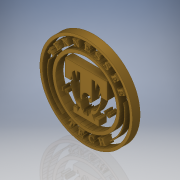
# Autodesk Inventor part: Brass Logo
Saved by Autodesk Inventor 2018 (Build 220112000, 112)
## iProperties
Created: 2017-11-28
Part Number: Brass Logo
Material: Brass, Soft Yellow
Document SubType Name: Modeling
Designer: Rus
Density: 8.47 g/cm^3
Appearance: Brass - Satin
Author: Rus
Autodesk Inventor part; units mm, degrees
(part 1 of 4)
ref_plane "YZ Plane" through (0, 0, 0) normal (1, 0, 0) x (0, 1, 0)
ref_plane "XZ Plane" through (0, 0, 0) normal (0, 1, 0) x (-1, 0, 0)
ref_plane "XY Plane" through (0, 0, 0) normal (0, 0, 1) x (1, 0, 0)
sketch "Sketch1" plane through (0, 0, 0) normal (0, 0, 1) x (1, 0, 0)
  line L0 (3.701247, -2.541841) -> (-3.701247, -2.541841)
  arc A0 (-5.715, -0.528088) -> (-3.701247, -2.541841) centre (-3.701247, -0.528088) ccw
  spline S0 degree 4 poles (-5.715, -0.528088) (-5.715, 3.281347) (0, 6.58346) (5.715, 3.281347) (5.715, -0.528088) knots -1 -1 -1 -1 -1 0 0 0 0 0
  arc A1 (3.701247, -2.541841) -> (5.715, -0.528088) centre (3.701247, -0.528088) ccw
  line L1 (9.525, -4.925915) -> (9.525, -1.750915)
  spline S1 degree 4 poles (9.525, -1.750915) (9.525, 7.774085) (0, 7.774085) (-9.525, 7.774085) (-9.525, -1.750915) knots 1 1 1 1 1 2 2 2 2 2
  line L2 (-9.525, -1.750915) -> (-9.525, -4.925915)
  arc A2 (-9.525, -4.925915) -> (9.525, -4.925915) centre (0, -45.086841) ccw
  circle A3 centre (0, -45.086841) radius 38.1
  dimension "d0" = 76.2
  constraints: 1 centre point, 1 coincident
  measures "d0" diameter of A3
extrude "Extrusion1" add sketch "Sketch1" along normal mid plane 6.35 contours A3
sketch "Sketch3" plane through (0, -45.086841, 3.175) normal (0, 0, 1) x (1, 0, 0)
  line L0 (0, -35.952322) -> (-0.919924, -35.952322)
  line L1 (-0.919924, -35.952322) -> (-3.676459, -35.766299)
  line L2 (-3.676459, -35.766299) -> (-7.246239, -35.221621)
  line L3 (-7.246239, -35.221621) -> (-10.691812, -34.335872)
  line L4 (-10.691812, -34.335872) -> (-13.995083, -33.126655)
  line L5 (-13.995083, -33.126655) -> (-17.136999, -31.612542)
  line L6 (-17.136999, -31.612542) -> (-20.101103, -29.812145)
  line L7 (-20.101103, -29.812145) -> (-22.868896, -27.741982)
  line L8 (-22.868896, -27.741982) -> (-25.421692, -25.421692)
  line L9 (-25.421692, -25.421692) -> (-27.74301, -22.868896)
  line L10 (-27.74301, -22.868896) -> (-29.812145, -20.101103)
  line L11 (-29.812145, -20.101103) -> (-31.612542, -17.136999)
  line L12 (-31.612542, -17.136999) -> (-33.126655, -13.99394)
  line L13 (-33.126655, -13.99394) -> (-34.335872, -10.690669)
  line L14 (-34.335872, -10.690669) -> (-35.221621, -7.246239)
  line L15 (-35.221621, -7.246239) -> (-35.766299, -3.67646)
  line L16 (-35.766299, -3.67646) -> (-35.951293, -0.919925)
  line L17 (-35.951293, -0.919925) -> (-35.951293, -0.001143)
  line L18 (-35.951293, -0.001143) -> (-35.951293, 0.918972)
  line L19 (-35.951293, 0.918972) -> (-35.766299, 3.675316)
  line L20 (-35.766299, 3.675316) -> (-35.221621, 7.245096)
  line L21 (-35.221621, 7.245096) -> (-34.335872, 10.689717)
  line L22 (-34.335872, 10.689717) -> (-33.126655, 13.992987)
  line L23 (-33.126655, 13.992987) -> (-31.612542, 17.136046)
  line L24 (-31.612542, 17.136046) -> (-29.812145, 20.100036)
  line L25 (-29.812145, 20.100036) -> (-27.74301, 22.868001)
  line L26 (-27.74301, 22.868001) -> (-25.421692, 25.420701)
  line L27 (-25.421692, 25.420701) -> (-22.868896, 27.740991)
  line L28 (-22.868896, 27.740991) -> (-20.101103, 29.811155)
  line L29 (-20.101103, 29.811155) -> (-17.136999, 31.61157)
  line L30 (-17.136999, 31.61157) -> (-13.995083, 33.125664)
  line L31 (-13.995083, 33.125664) -> (-10.691812, 34.334958)
  line L32 (-10.691812, 34.334958) -> (-7.246239, 35.220592)
  line L33 (-7.246239, 35.220592) -> (-3.676459, 35.765232)
  line L34 (-3.676459, 35.765232) -> (-0.919924, 35.950207)
  line L35 (-0.919924, 35.950207) -> (0, 35.950207)
  line L36 (0, 35.950207) -> (0.918972, 35.950207)
  line L37 (0.918972, 35.950207) -> (3.675317, 35.765232)
  line L38 (3.675317, 35.765232) -> (7.245096, 35.220592)
  line L39 (7.245096, 35.220592) -> (10.69067, 34.334958)
  line L40 (10.69067, 34.334958) -> (13.99413, 33.125664)
  line L41 (13.99413, 33.125664) -> (17.136999, 31.61157)
  line L42 (17.136999, 31.61157) -> (20.101179, 29.811155)
  line L43 (20.101179, 29.811155) -> (22.868954, 27.740991)
  line L44 (22.868954, 27.740991) -> (25.421653, 25.420701)
  line L45 (25.421653, 25.420701) -> (27.742134, 22.868001)
  line L46 (27.742134, 22.868001) -> (29.812107, 20.100036)
  line L47 (29.812107, 20.100036) -> (31.612332, 17.136046)
  line L48 (31.612332, 17.136046) -> (33.126617, 13.992987)
  line L49 (33.126617, 13.992987) -> (34.33572, 10.689717)
  line L50 (34.33572, 10.689717) -> (35.221545, 7.245096)
  line L51 (35.221545, 7.245096) -> (35.766375, 3.675316)
  line L52 (35.766375, 3.675316) -> (35.952303, 0.918972)
  line L53 (35.952303, 0.918972) -> (35.952303, -0.001143)
  line L54 (35.952303, -0.001143) -> (35.952303, -0.919925)
  line L55 (35.952303, -0.919925) -> (35.766375, -3.67646)
  line L56 (35.766375, -3.67646) -> (35.221545, -7.246239)
  line L57 (35.221545, -7.246239) -> (34.33572, -10.690669)
  line L58 (34.33572, -10.690669) -> (33.126617, -13.99394)
  line L59 (33.126617, -13.99394) -> (31.612332, -17.136999)
  line L60 (31.612332, -17.136999) -> (29.812107, -20.101103)
  line L61 (29.812107, -20.101103) -> (27.742134, -22.868896)
  line L62 (27.742134, -22.868896) -> (25.421653, -25.421692)
  line L63 (25.421653, -25.421692) -> (22.868954, -27.741982)
  line L64 (22.868954, -27.741982) -> (20.101179, -29.812145)
  line L65 (20.101179, -29.812145) -> (17.136999, -31.612542)
  line L66 (17.136999, -31.612542) -> (13.99413, -33.126655)
  line L67 (13.99413, -33.126655) -> (10.69067, -34.335872)
  line L68 (10.69067, -34.335872) -> (7.245096, -35.221621)
  line L69 (7.245096, -35.221621) -> (3.675317, -35.766299)
  line L70 (3.675317, -35.766299) -> (0.918972, -35.952322)
  line L71 (0.918972, -35.952322) -> (0, -35.952322)
  line L72 (0, 38.098857) -> (-0.974788, 38.098857)
  line L73 (-0.974788, 38.098857) -> (-3.896487, 37.902642)
  line L74 (-3.896487, 37.902642) -> (-7.679055, 37.325808)
  line L75 (-7.679055, 37.325808) -> (-11.330559, 36.386262)
  line L76 (-11.330559, 36.386262) -> (-14.830044, 35.104959)
  line L77 (-14.830044, 35.104959) -> (-18.161127, 33.500758)
  line L78 (-18.161127, 33.500758) -> (-21.302053, 31.592901)
  line L79 (-21.302053, 31.592901) -> (-24.235219, 29.398722)
  line L80 (-24.235219, 29.398722) -> (-26.940986, 26.939938)
  line L81 (-26.940986, 26.939938) -> (-29.399751, 24.234267)
  line L82 (-29.399751, 24.234267) -> (-31.593949, 21.301138)
  line L83 (-31.593949, 21.301138) -> (-33.501825, 18.160174)
  line L84 (-33.501825, 18.160174) -> (-35.105873, 14.829091)
  line L85 (-35.105873, 14.829091) -> (-36.387441, 11.329416)
  line L86 (-36.387441, 11.329416) -> (-37.326919, 7.678293)
  line L87 (-37.326919, 7.678293) -> (-37.903629, 3.895534)
  line L88 (-37.903629, 3.895534) -> (-38.1, 0.973645)
  line L89 (-38.1, 0.973645) -> (-38.1, -0.001143)
  line L90 (-38.1, -0.001143) -> (-38.1, -0.974789)
  line L91 (-38.1, -0.974789) -> (-37.903629, -3.896487)
  line L92 (-37.903629, -3.896487) -> (-37.326919, -7.679055)
  line L93 (-37.326919, -7.679055) -> (-36.387441, -11.329416)
  line L94 (-36.387441, -11.329416) -> (-35.105873, -14.830044)
  line L95 (-35.105873, -14.830044) -> (-33.501825, -18.161127)
  line L96 (-33.501825, -18.161127) -> (-31.593949, -21.302053)
  line L97 (-31.593949, -21.302053) -> (-29.399751, -24.23522)
  line L98 (-29.399751, -24.23522) -> (-26.940986, -26.940986)
  line L99 (-26.940986, -26.940986) -> (-24.235219, -29.399751)
  line L100 (-24.235219, -29.399751) -> (-21.302053, -31.592882)
  line L101 (-21.302053, -31.592882) -> (-18.161127, -33.500797)
  line L102 (-18.161127, -33.500797) -> (-14.830044, -35.105873)
  line L103 (-14.830044, -35.105873) -> (-11.330559, -36.386411)
  line L104 (-11.330559, -36.386411) -> (-7.679055, -37.325888)
  line L105 (-7.679055, -37.325888) -> (-3.896487, -37.902596)
  line L106 (-3.896487, -37.902596) -> (-0.974788, -38.1)
  line L107 (-0.974788, -38.1) -> (0, -38.1)
  line L108 (0, -38.1) -> (0.973645, -38.1)
  line L109 (0.973645, -38.1) -> (3.895535, -37.902596)
  line L110 (3.895535, -37.902596) -> (7.678293, -37.325888)
  line L111 (7.678293, -37.325888) -> (11.329416, -36.386411)
  line L112 (11.329416, -36.386411) -> (14.829091, -35.105873)
  line L113 (14.829091, -35.105873) -> (18.160175, -33.500797)
  line L114 (18.160175, -33.500797) -> (21.301139, -31.592882)
  line L115 (21.301139, -31.592882) -> (24.234267, -29.399751)
  line L116 (24.234267, -29.399751) -> (26.939939, -26.940986)
  line L117 (26.939939, -26.940986) -> (29.398722, -24.23522)
  line L118 (29.398722, -24.23522) -> (31.592901, -21.302053)
  line L119 (31.592901, -21.302053) -> (33.500758, -18.161127)
  line L120 (33.500758, -18.161127) -> (35.104959, -14.830044)
  line L121 (35.104959, -14.830044) -> (36.386262, -11.329416)
  line L122 (36.386262, -11.329416) -> (37.325808, -7.679055)
  line L123 (37.325808, -7.679055) -> (37.902642, -3.896487)
  line L124 (37.902642, -3.896487) -> (38.1, -0.974789)
  line L125 (38.1, -0.974789) -> (38.1, -0.001143)
  line L126 (38.1, -0.001143) -> (38.1, 0.973645)
  line L127 (38.1, 0.973645) -> (37.902642, 3.895534)
  line L128 (37.902642, 3.895534) -> (37.325808, 7.678293)
  line L129 (37.325808, 7.678293) -> (36.386262, 11.329416)
  line L130 (36.386262, 11.329416) -> (35.104959, 14.829091)
  line L131 (35.104959, 14.829091) -> (33.500758, 18.160174)
  line L132 (33.500758, 18.160174) -> (31.592901, 21.301138)
  line L133 (31.592901, 21.301138) -> (29.398722, 24.234267)
  line L134 (29.398722, 24.234267) -> (26.939939, 26.939938)
  line L135 (26.939939, 26.939938) -> (24.234267, 29.398722)
  line L136 (24.234267, 29.398722) -> (21.301139, 31.592901)
  line L137 (21.301139, 31.592901) -> (18.160175, 33.500758)
  line L138 (18.160175, 33.500758) -> (14.829091, 35.104959)
  line L139 (14.829091, 35.104959) -> (11.329416, 36.386262)
  line L140 (11.329416, 36.386262) -> (7.678293, 37.325808)
  line L141 (7.678293, 37.325808) -> (3.895535, 37.902642)
  line L142 (3.895535, 37.902642) -> (0.973645, 38.098857)
  line L143 (0.973645, 38.098857) -> (0, 38.098857)
  line L144 (0, -25.161259) -> (-1.268158, -25.161259)
  line L145 (-1.268158, -25.161259) -> (-5.071491, -24.649671)
  line L146 (-5.071491, -24.649671) -> (-9.794938, -23.183088)
  line L147 (-9.794938, -23.183088) -> (-14.068425, -20.863846)
  line L148 (-14.068425, -20.863846) -> (-17.792128, -17.791176)
  line L149 (-17.792128, -17.791176) -> (-20.864874, -14.068425)
  line L150 (-20.864874, -14.068425) -> (-23.184117, -9.793796)
  line L151 (-23.184117, -9.793796) -> (-24.6507, -5.071491)
  line L152 (-24.6507, -5.071491) -> (-25.161259, -1.268159)
  line L153 (-25.161259, -1.268159) -> (-25.161259, -0.001143)
  line L154 (-25.161259, -0.001143) -> (-25.161259, 1.267015)
  line L155 (-25.161259, 1.267015) -> (-24.6507, 5.070538)
  line L156 (-24.6507, 5.070538) -> (-23.184117, 9.793795)
  line L157 (-23.184117, 9.793795) -> (-20.864874, 14.067282)
  line L158 (-20.864874, 14.067282) -> (-17.792128, 17.791176)
  line L159 (-17.792128, 17.791176) -> (-14.068425, 20.86375)
  line L160 (-14.068425, 20.86375) -> (-9.794938, 23.183088)
  line L161 (-9.794938, 23.183088) -> (-5.071491, 24.649557)
  line L162 (-5.071491, 24.649557) -> (-1.268158, 25.160287)
  line L163 (-1.268158, 25.160287) -> (0, 25.160287)
  line L164 (0, 25.160287) -> (1.267016, 25.160287)
  line L165 (1.267016, 25.160287) -> (5.070539, 24.649557)
  line L166 (5.070539, 24.649557) -> (9.793795, 23.183088)
  line L167 (9.793795, 23.183088) -> (14.067282, 20.86375)
  line L168 (14.067282, 20.86375) -> (17.791176, 17.791176)
  line L169 (17.791176, 17.791176) -> (20.86375, 14.067282)
  line L170 (20.86375, 14.067282) -> (23.183088, 9.793795)
  line L171 (23.183088, 9.793795) -> (24.649557, 5.070538)
  line L172 (24.649557, 5.070538) -> (25.161431, 1.267015)
  line L173 (25.161431, 1.267015) -> (25.161431, -0.001143)
  line L174 (25.161431, -0.001143) -> (25.161431, -1.268159)
  line L175 (25.161431, -1.268159) -> (24.649557, -5.071491)
  line L176 (24.649557, -5.071491) -> (23.183088, -9.793796)
  line L177 (23.183088, -9.793796) -> (20.86375, -14.068425)
  line L178 (20.86375, -14.068425) -> (17.791176, -17.791176)
  line L179 (17.791176, -17.791176) -> (14.067282, -20.863846)
  line L180 (14.067282, -20.863846) -> (9.793795, -23.183088)
  line L181 (9.793795, -23.183088) -> (5.070539, -24.649671)
  line L182 (5.070539, -24.649671) -> (1.267016, -25.161259)
  line L183 (1.267016, -25.161259) -> (0, -25.161259)
  line L184 (0, 27.596211) -> (-0.705993, 27.596211)
  line L185 (-0.705993, 27.596211) -> (-2.822638, 27.454669)
  line L186 (-2.822638, 27.454669) -> (-5.562409, 27.036141)
  line L187 (-5.562409, 27.036141) -> (-8.207311, 26.355866)
  line L188 (-8.207311, 26.355866) -> (-10.742676, 25.427749)
  line L189 (-10.742676, 25.427749) -> (-13.154787, 24.266271)
  line L190 (-13.154787, 24.266271) -> (-15.4305, 22.883241)
  line L191 (-15.4305, 22.883241) -> (-17.554575, 21.294661)
  line L192 (-17.554575, 21.294661) -> (-19.515087, 19.514058)
  line L193 (-19.515087, 19.514058) -> (-21.295862, 17.553432)
  line L194 (-21.295862, 17.553432) -> (-22.884403, 15.429357)
  line L195 (-22.884403, 15.429357) -> (-24.267243, 13.153834)
  line L196 (-24.267243, 13.153834) -> (-25.42895, 10.741533)
  line L197 (-25.42895, 10.741533) -> (-26.357047, 8.206359)
  line L198 (-26.357047, 8.206359) -> (-27.037113, 5.561457)
  line L199 (-27.037113, 5.561457) -> (-27.455679, 2.821495)
  line L200 (-27.455679, 2.821495) -> (-27.597278, 0.70485)
  line L201 (-27.597278, 0.70485) -> (-27.597278, -0.001143)
  line L202 (-27.597278, -0.001143) -> (-27.597278, -0.705993)
  line L203 (-27.597278, -0.705993) -> (-27.455679, -2.821496)
  line L204 (-27.455679, -2.821496) -> (-27.037113, -5.56241)
  line L205 (-27.037113, -5.56241) -> (-26.357047, -8.206359)
  line L206 (-26.357047, -8.206359) -> (-25.42895, -10.742676)
  line L207 (-25.42895, -10.742676) -> (-24.267243, -13.154787)
  line L208 (-24.267243, -13.154787) -> (-22.884403, -15.429547)
  line L209 (-22.884403, -15.429547) -> (-21.295862, -17.554575)
  line L210 (-21.295862, -17.554575) -> (-19.515087, -19.514058)
  line L211 (-19.515087, -19.514058) -> (-17.554575, -21.294833)
  line L212 (-17.554575, -21.294833) -> (-15.4305, -22.883355)
  line L213 (-15.4305, -22.883355) -> (-13.154787, -24.266214)
  line L214 (-13.154787, -24.266214) -> (-10.742676, -25.427921)
  line L215 (-10.742676, -25.427921) -> (-8.207311, -26.356018)
  line L216 (-8.207311, -26.356018) -> (-5.562409, -27.036084)
  line L217 (-5.562409, -27.036084) -> (-2.822638, -27.45465)
  line L218 (-2.822638, -27.45465) -> (-0.705993, -27.597278)
  line L219 (-0.705993, -27.597278) -> (0, -27.597278)
  line L220 (0, -27.597278) -> (0.70485, -27.597278)
  line L221 (0.70485, -27.597278) -> (2.821496, -27.45465)
  line L222 (2.821496, -27.45465) -> (5.561457, -27.036084)
  line L223 (5.561457, -27.036084) -> (8.206359, -26.356018)
  line L224 (8.206359, -26.356018) -> (10.741533, -25.427921)
  line L225 (10.741533, -25.427921) -> (13.153835, -24.266214)
  line L226 (13.153835, -24.266214) -> (15.429357, -22.883355)
  line L227 (15.429357, -22.883355) -> (17.553432, -21.294833)
  line L228 (17.553432, -21.294833) -> (19.514058, -19.514058)
  line L229 (19.514058, -19.514058) -> (21.294662, -17.554575)
  line L230 (21.294662, -17.554575) -> (22.883241, -15.429547)
  line L231 (22.883241, -15.429547) -> (24.266271, -13.154787)
  line L232 (24.266271, -13.154787) -> (25.42775, -10.742676)
  line L233 (25.42775, -10.742676) -> (26.355866, -8.206359)
  line L234 (26.355866, -8.206359) -> (27.036141, -5.56241)
  line L235 (27.036141, -5.56241) -> (27.454669, -2.821496)
  line L236 (27.454669, -2.821496) -> (27.597354, -0.705993)
  line L237 (27.597354, -0.705993) -> (27.597354, -0.001143)
  line L238 (27.597354, -0.001143) -> (27.597354, 0.70485)
  line L239 (27.597354, 0.70485) -> (27.454669, 2.821495)
  line L240 (27.454669, 2.821495) -> (27.036141, 5.561457)
  line L241 (27.036141, 5.561457) -> (26.355866, 8.206359)
  line L242 (26.355866, 8.206359) -> (25.42775, 10.741533)
  line L243 (25.42775, 10.741533) -> (24.266271, 13.153834)
  line L244 (24.266271, 13.153834) -> (22.883241, 15.429357)
  line L245 (22.883241, 15.429357) -> (21.294662, 17.553432)
  line L246 (21.294662, 17.553432) -> (19.514058, 19.514058)
  line L247 (19.514058, 19.514058) -> (17.553432, 21.294661)
  line L248 (17.553432, 21.294661) -> (15.429357, 22.883241)
  line L249 (15.429357, 22.883241) -> (13.153835, 24.266271)
  line L250 (13.153835, 24.266271) -> (10.741533, 25.427749)
  line L251 (10.741533, 25.427749) -> (8.206359, 26.355866)
  line L252 (8.206359, 26.355866) -> (5.561457, 27.036141)
  line L253 (5.561457, 27.036141) -> (2.821496, 27.454669)
  line L254 (2.821496, 27.454669) -> (0.70485, 27.596211)
  line L255 (0.70485, 27.596211) -> (0, 27.596211)
  line L256 (17.172051, 16.11268) -> (17.172051, 2.422588)
  line L257 (17.172051, 2.422588) -> (12.363259, 2.422588)
  line L258 (12.363259, 2.422588) -> (12.363259, 2.817304)
  line L259 (12.363259, 2.817304) -> (12.3063, 3.999738)
  line L260 (12.3063, 3.999738) -> (12.175045, 5.195697)
  line L261 (12.175045, 5.195697) -> (12.137708, 5.418582)
  line L262 (12.137708, 5.418582) -> (9.773222, 1.311592)
  line L263 (9.773222, 1.311592) -> (11.41838, 8.127682)
  line L264 (11.41838, 8.127682) -> (11.292459, 8.4201)
  line L265 (11.292459, 8.4201) -> (10.479786, 9.628441)
  line L266 (10.479786, 9.628441) -> (9.415463, 10.516171)
  line L267 (9.415463, 10.516171) -> (9.16324, 10.648378)
  line L268 (9.16324, 10.648378) -> (7.332916, 4.981575)
  line L269 (7.332916, 4.981575) -> (7.258621, 11.266551)
  line L270 (7.258621, 11.266551) -> (7.070407, 11.299507)
  line L271 (7.070407, 11.299507) -> (6.058472, 11.397805)
  line L272 (6.058472, 11.397805) -> (4.950524, 11.415522)
  line L273 (4.950524, 11.415522) -> (4.714875, 11.406949)
  line L274 (4.714875, 11.406949) -> (4.725162, -4.028885)
  line L275 (4.725162, -4.028885) -> (4.725162, -4.259199)
  line L276 (4.725162, -4.259199) -> (4.528947, -4.953762)
  line L277 (4.528947, -4.953762) -> (4.022408, -5.571935)
  line L278 (4.022408, -5.571935) -> (3.332226, -5.801296)
  line L279 (3.332226, -5.801296) -> (2.736914, -5.668899)
  line L280 (2.736914, -5.668899) -> (2.579751, -5.564505)
  line L281 (2.579751, -5.564505) -> (2.432876, -5.466207)
  line L282 (2.432876, -5.466207) -> (2.098167, -5.013579)
  line L283 (2.098167, -5.013579) -> (1.903667, -4.272534)
  line L284 (1.903667, -4.272534) -> (2.051495, -3.487293)
  line L285 (2.051495, -3.487293) -> (2.427732, -2.934272)
  line L286 (2.427732, -2.934272) -> (2.596325, -2.805875)
  line L287 (2.596325, -2.805875) -> (3.382709, -2.657285)
  line L288 (3.382709, -2.657285) -> (3.809429, -2.90322)
  line L289 (3.809429, -2.90322) -> (3.837432, -2.702624)
  line L290 (3.837432, -2.702624) -> (3.792093, -2.084642)
  line L291 (3.792093, -2.084642) -> (3.49758, -1.562672)
  line L292 (3.49758, -1.562672) -> (2.978658, -1.279589)
  line L293 (2.978658, -1.279589) -> (2.462022, -1.185291)
  line L294 (2.462022, -1.185291) -> (2.289239, -1.179195)
  line L295 (2.289239, -1.179195) -> (2.020633, -1.011746)
  line L296 (2.020633, -1.011746) -> (1.109853, -0.676085)
  line L297 (1.109853, -0.676085) -> (-0.02267, -0.608838)
  line L298 (-0.02267, -0.608838) -> (-1.061466, -0.920687)
  line L299 (-1.061466, -0.920687) -> (-1.959483, -1.555433)
  line L300 (-1.959483, -1.555433) -> (-2.670619, -2.454593)
  line L301 (-2.670619, -2.454593) -> (-3.148012, -3.562541)
  line L302 (-3.148012, -3.562541) -> (-3.344608, -4.820412)
  line L303 (-3.344608, -4.820412) -> (-3.287649, -5.843588)
  line L304 (-3.287649, -5.843588) -> (-3.213354, -6.1722)
  line L305 (-3.213354, -6.1722) -> (-3.182112, -6.310884)
  line L306 (-3.182112, -6.310884) -> (-3.203829, -6.785229)
  line L307 (-3.203829, -6.785229) -> (-3.458146, -7.027926)
  line L308 (-3.458146, -7.027926) -> (-3.54311, -7.050596)
  line L309 (-3.54311, -7.050596) -> (-3.686746, -7.087934)
  line L310 (-3.686746, -7.087934) -> (-4.161854, -7.030974)
  line L311 (-4.161854, -7.030974) -> (-4.604194, -6.670358)
  line L312 (-4.604194, -6.670358) -> (-4.868799, -6.078284)
  line L313 (-4.868799, -6.078284) -> (-4.95662, -5.54374)
  line L314 (-4.95662, -5.54374) -> (-4.95662, -5.366004)
  line L315 (-4.95662, -5.366004) -> (-4.946332, 11.406949)
  line L316 (-4.946332, 11.406949) -> (-5.183124, 11.415522)
  line L317 (-5.183124, 11.415522) -> (-6.291072, 11.397805)
  line L318 (-6.291072, 11.397805) -> (-7.302055, 11.298555)
  line L319 (-7.302055, 11.298555) -> (-7.490079, 11.265408)
  line L320 (-7.490079, 11.265408) -> (-7.564374, 4.981575)
  line L321 (-7.564374, 4.981575) -> (-9.394889, 10.648378)
  line L322 (-9.394889, 10.648378) -> (-9.64692, 10.516171)
  line L323 (-9.64692, 10.516171) -> (-10.711434, 9.628441)
  line L324 (-10.711434, 9.628441) -> (-11.522964, 8.418957)
  line L325 (-11.522964, 8.418957) -> (-11.648884, 8.12673)
  line L326 (-11.648884, 8.12673) -> (-10.004488, 1.311592)
  line L327 (-10.004488, 1.311592) -> (-12.356782, 5.399151)
  line L328 (-12.356782, 5.399151) -> (-12.395073, 5.176837)
  line L329 (-12.395073, 5.176837) -> (-12.528423, 3.988308)
  line L330 (-12.528423, 3.988308) -> (-12.584239, 2.814447)
  line L331 (-12.584239, 2.814447) -> (-12.584239, 2.422588)
  line L332 (-12.584239, 2.422588) -> (-17.341596, 2.422588)
  line L333 (-17.341596, 2.422588) -> (-17.341596, 16.11268)
  line L334 (-17.341596, 16.11268) -> (17.172051, 16.11268)
  line L335 (1.435608, -12.052935) -> (2.963037, -14.304074)
  line L336 (2.963037, -14.304074) -> (3.054096, -14.131481)
  line L337 (3.054096, -14.131481) -> (3.477959, -13.134022)
  line L338 (3.477959, -13.134022) -> (3.854958, -11.942445)
  line L339 (3.854958, -11.942445) -> (3.923157, -11.673649)
  line L340 (3.923157, -11.673649) -> (4.728401, -9.001125)
  line L341 (4.728401, -9.001125) -> (4.776978, -9.177528)
  line L342 (4.776978, -9.177528) -> (5.028057, -9.683305)
  line L343 (5.028057, -9.683305) -> (5.437442, -10.062401)
  line L344 (5.437442, -10.062401) -> (5.922074, -10.187559)
  line L345 (5.922074, -10.187559) -> (6.446139, -10.110026)
  line L346 (6.446139, -10.110026) -> (6.974205, -9.877425)
  line L347 (6.974205, -9.877425) -> (7.470267, -9.540621)
  line L348 (7.470267, -9.540621) -> (7.900225, -9.149906)
  line L349 (7.900225, -9.149906) -> (8.155495, -8.85825)
  line L350 (8.155495, -8.85825) -> (8.229029, -8.754047)
  line L351 (8.229029, -8.754047) -> (8.690039, -8.088249)
  line L352 (8.690039, -8.088249) -> (9.885616, -5.960174)
  line L353 (9.885616, -5.960174) -> (11.095101, -3.139821)
  line L354 (11.095101, -3.139821) -> (11.871008, -0.474345)
  line L355 (11.871008, -0.474345) -> (12.186475, 1.269111)
  line L356 (12.186475, 1.269111) -> (12.228766, 1.854136)
  line L357 (12.228766, 1.854136) -> (12.233719, 1.745742)
  line L358 (12.233719, 1.745742) -> (12.257532, 0.599503)
  line L359 (12.257532, 0.599503) -> (12.257532, 0.478726)
  line L360 (12.257532, 0.478726) -> (12.255437, -0.115634)
  line L361 (12.255437, -0.115634) -> (12.008549, -1.901571)
  line L362 (12.008549, -1.901571) -> (11.267504, -4.741926)
  line L363 (11.267504, -4.741926) -> (10.014014, -7.805166)
  line L364 (10.014014, -7.805166) -> (8.731187, -10.131743)
  line L365 (8.731187, -10.131743) -> (8.229029, -10.856024)
  line L366 (8.229029, -10.856024) -> (8.162925, -10.950321)
  line L367 (8.162925, -10.950321) -> (7.954137, -11.226356)
  line L368 (7.954137, -11.226356) -> (7.590282, -11.667554)
  line L369 (7.590282, -11.667554) -> (7.162228, -12.131611)
  line L370 (7.162228, -12.131611) -> (6.693217, -12.57281)
  line L371 (6.693217, -12.57281) -> (6.208395, -12.941808)
  line L372 (6.208395, -12.941808) -> (5.731955, -13.193078)
  line L373 (5.731955, -13.193078) -> (5.287518, -13.278802)
  line L374 (5.287518, -13.278802) -> (4.978337, -13.207555)
  line L375 (4.978337, -13.207555) -> (4.900041, -13.151739)
  line L376 (4.900041, -13.151739) -> (4.910328, -13.227177)
  line L377 (4.910328, -13.227177) -> (5.110734, -13.861732)
  line L378 (5.110734, -13.861732) -> (5.144834, -13.927836)
  line L379 (5.144834, -13.927836) -> (6.803707, -17.177195)
  line L380 (6.803707, -17.177195) -> (6.803707, -14.610017)
  line L381 (6.803707, -14.610017) -> (6.829615, -14.613065)
  line L382 (6.829615, -14.613065) -> (7.101459, -14.645069)
  line L383 (7.101459, -14.645069) -> (7.130224, -14.648117)
  line L384 (7.130224, -14.648117) -> (7.284339, -14.665833)
  line L385 (7.284339, -14.665833) -> (8.410765, -14.740128)
  line L386 (8.410765, -14.740128) -> (10.014966, -14.79804)
  line L387 (10.014966, -14.79804) -> (10.407586, -14.807375)
  line L388 (10.407586, -14.807375) -> (10.407586, -19.352819)
  line L389 (10.407586, -19.352819) -> (-10.628757, -19.352819)
  line L390 (-10.628757, -19.352819) -> (-10.628757, -14.807375)
  line L391 (-10.628757, -14.807375) -> (-10.244328, -14.807375)
  line L392 (-10.244328, -14.807375) -> (-9.089707, -14.779371)
  line L393 (-9.089707, -14.779371) -> (-7.975854, -14.712315)
  line L394 (-7.975854, -14.712315) -> (-7.775257, -14.692694)
  line L395 (-7.775257, -14.692694) -> (-7.705915, -14.685454)
  line L396 (-7.705915, -14.685454) -> (-7.051738, -14.602778)
  line L397 (-7.051738, -14.602778) -> (-6.990779, -14.593443)
  line L398 (-6.990779, -14.593443) -> (-6.990779, -17.177195)
  line L399 (-6.990779, -17.177195) -> (-5.38372, -14.030135)
  line L400 (-5.38372, -14.030135) -> (-5.346383, -13.955649)
  line L401 (-5.346383, -13.955649) -> (-5.071491, -13.174409)
  line L402 (-5.071491, -13.174409) -> (-5.060061, -13.094779)
  line L403 (-5.060061, -13.094779) -> (-5.134546, -13.162026)
  line L404 (-5.134546, -13.162026) -> (-5.443537, -13.272516)
  line L405 (-5.443537, -13.272516) -> (-5.892355, -13.217843)
  line L406 (-5.892355, -13.217843) -> (-6.377749, -12.982194)
  line L407 (-6.377749, -12.982194) -> (-6.874955, -12.614148)
  line L408 (-6.874955, -12.614148) -> (-7.358634, -12.167807)
  line L409 (-7.358634, -12.167807) -> (-7.802118, -11.691366)
  line L410 (-7.802118, -11.691366) -> (-8.177212, -11.236642)
  line L411 (-8.177212, -11.236642) -> (-8.392287, -10.953179)
  line L412 (-8.392287, -10.953179) -> (-8.459533, -10.856024)
  line L413 (-8.459533, -10.856024) -> (-8.961691, -10.131743)
  line L414 (-8.961691, -10.131743) -> (-10.245471, -7.805166)
  line L415 (-10.245471, -7.805166) -> (-11.498961, -4.741926)
  line L416 (-11.498961, -4.741926) -> (-12.241149, -1.901571)
  line L417 (-12.241149, -1.901571) -> (-12.487084, -0.115634)
  line L418 (-12.487084, -0.115634) -> (-12.48918, 0.478726)
  line L419 (-12.48918, 0.478726) -> (-12.490132, 0.599503)
  line L420 (-12.490132, 0.599503) -> (-12.465367, 1.745742)
  line L421 (-12.465367, 1.745742) -> (-12.459081, 1.854136)
  line L422 (-12.459081, 1.854136) -> (-12.41679, 1.269111)
  line L423 (-12.41679, 1.269111) -> (-12.102655, -0.474345)
  line L424 (-12.102655, -0.474345) -> (-11.326558, -3.139821)
  line L425 (-11.326558, -3.139821) -> (-10.117074, -5.960174)
  line L426 (-10.117074, -5.960174) -> (-8.921496, -8.088249)
  line L427 (-8.921496, -8.088249) -> (-8.459533, -8.754047)
  line L428 (-8.459533, -8.754047) -> (-8.386953, -8.85825)
  line L429 (-8.386953, -8.85825) -> (-8.132826, -9.149906)
  line L430 (-8.132826, -9.149906) -> (-7.702867, -9.540621)
  line L431 (-7.702867, -9.540621) -> (-7.205662, -9.877425)
  line L432 (-7.205662, -9.877425) -> (-6.678549, -10.110026)
  line L433 (-6.678549, -10.110026) -> (-6.154674, -10.187559)
  line L434 (-6.154674, -10.187559) -> (-5.670042, -10.062401)
  line L435 (-5.670042, -10.062401) -> (-5.259705, -9.683305)
  line L436 (-5.259705, -9.683305) -> (-5.007483, -9.178671)
  line L437 (-5.007483, -9.178671) -> (-4.958905, -9.001125)
  line L438 (-4.958905, -9.001125) -> (-4.153662, -11.673649)
  line L439 (-4.153662, -11.673649) -> (-4.082605, -11.956923)
  line L440 (-4.082605, -11.956923) -> (-3.681412, -13.206412)
  line L441 (-3.681412, -13.206412) -> (-3.227641, -14.241018)
  line L442 (-3.227641, -14.241018) -> (-3.129534, -14.417802)
  line L443 (-3.129534, -14.417802) -> (-1.523429, -12.052935)
  line L444 (-1.523429, -12.052935) -> (-2.357437, -15.50289)
  line L445 (-2.357437, -15.50289) -> (-2.234375, -15.635288)
  line L446 (-2.234375, -15.635288) -> (-1.584388, -16.134398)
  line L447 (-1.584388, -16.134398) -> (-0.900112, -16.433102)
  line L448 (-0.900112, -16.433102) -> (-0.758571, -16.465106)
  line L449 (-0.758571, -16.465106) -> (-0.027813, -12.36726)
  line L450 (-0.027813, -12.36726) -> (0.783336, -16.399002)
  line L451 (0.783336, -16.399002) -> (0.911543, -16.356711)
  line L452 (0.911543, -16.356711) -> (1.534859, -16.02486)
  line L453 (1.534859, -16.02486) -> (2.126933, -15.51432)
  line L454 (2.126933, -15.51432) -> (2.240661, -15.384018)
  line L455 (2.240661, -15.384018) -> (1.435608, -12.052935)
  line L456 (14.425803, -8.89235) -> (14.425803, -8.548497)
  line L457 (14.425803, -8.548497) -> (14.641068, -8.548497)
  line L458 (14.641068, -8.548497) -> (14.717458, -8.548497)
  line L459 (14.717458, -8.548497) -> (14.938629, -8.50392)
  line L460 (14.938629, -8.50392) -> (14.950059, -8.495538)
  line L461 (14.950059, -8.495538) -> (14.960346, -8.486203)
  line L462 (14.960346, -8.486203) -> (15.014067, -8.32085)
  line L463 (15.014067, -8.32085) -> (15.014067, -8.266176)
  line L464 (15.014067, -8.266176) -> (15.014067, -6.736461)
  line L465 (15.014067, -6.736461) -> (14.425803, -6.736461)
  line L466 (14.425803, -6.736461) -> (14.425803, -6.397562)
  line L467 (14.425803, -6.397562) -> (14.482763, -6.394514)
  line L468 (14.482763, -6.394514) -> (14.93158, -6.296216)
  line L469 (14.93158, -6.296216) -> (14.963585, -6.279642)
  line L470 (14.963585, -6.279642) -> (14.994445, -6.262116)
  line L471 (14.994445, -6.262116) -> (15.239428, -5.990463)
  line L472 (15.239428, -5.990463) -> (15.256954, -5.953125)
  line L473 (15.256954, -5.953125) -> (15.645575, -5.953125)
  line L474 (15.645575, -5.953125) -> (15.645575, -8.27532)
  line L475 (15.645575, -8.27532) -> (15.645575, -8.331136)
  line L476 (15.645575, -8.331136) -> (15.689009, -8.492681)
  line L477 (15.689009, -8.492681) -> (15.698343, -8.500872)
  line L478 (15.698343, -8.500872) -> (15.706535, -8.507921)
  line L479 (15.706535, -8.507921) -> (15.911322, -8.548497)
  line L480 (15.911322, -8.548497) -> (15.979521, -8.548497)
  line L481 (15.979521, -8.548497) -> (16.223171, -8.548497)
  line L482 (16.223171, -8.548497) -> (16.223171, -8.89235)
  line L483 (16.223171, -8.89235) -> (14.425803, -8.89235)
  line L484 (17.692878, -8.441817) -> (17.713643, -8.458391)
  line L485 (17.713643, -8.458391) -> (17.947196, -8.584311)
  line L486 (17.947196, -8.584311) -> (17.973104, -8.593646)
  line L487 (17.973104, -8.593646) -> (17.997678, -8.602218)
  line L488 (17.997678, -8.602218) -> (18.224183, -8.643366)
  line L489 (18.224183, -8.643366) -> (18.299621, -8.643366)
  line L490 (18.299621, -8.643366) -> (18.432018, -8.643366)
  line L491 (18.432018, -8.643366) -> (18.798921, -8.484108)
  line L492 (18.798921, -8.484108) -> (18.830925, -8.452104)
  line L493 (18.830925, -8.452104) -> (18.861977, -8.4201)
  line L494 (18.861977, -8.4201) -> (19.021235, -8.041957)
  line L495 (19.021235, -8.041957) -> (19.021235, -7.915846)
  line L496 (19.021235, -7.915846) -> (19.021235, -7.777353)
  line L497 (19.021235, -7.777353) -> (18.868263, -7.395972)
  line L498 (18.868263, -7.395972) -> (18.838164, -7.363968)
  line L499 (18.838164, -7.363968) -> (18.807113, -7.330821)
  line L500 (18.807113, -7.330821) -> (18.447639, -7.16642)
  line L501 (18.447639, -7.16642) -> (18.327624, -7.16642)
  line L502 (18.327624, -7.16642) -> (18.244947, -7.16642)
  line L503 (18.244947, -7.16642) -> (18.024729, -7.228332)
  line L504 (18.024729, -7.228332) -> (17.999964, -7.241858)
  line L505 (17.999964, -7.241858) -> (17.975199, -7.254431)
  line L506 (17.975199, -7.254431) -> (17.742789, -7.445692)
  line L507 (17.742789, -7.445692) -> (17.721072, -7.472363)
  line L508 (17.721072, -7.472363) -> (17.39627, -7.457885)
  line L509 (17.39627, -7.457885) -> (17.544288, -5.909691)
  line L510 (17.544288, -5.909691) -> (17.583341, -5.922264)
  line L511 (17.583341, -5.922264) -> (17.984534, -6.018276)
  line L512 (17.984534, -6.018276) -> (18.025872, -6.024563)
  line L513 (18.025872, -6.024563) -> (18.066068, -6.030659)
  line L514 (18.066068, -6.030659) -> (18.423636, -6.062663)
  line L515 (18.423636, -6.062663) -> (18.543651, -6.062663)
  line L516 (18.543651, -6.062663) -> (18.677953, -6.062663)
  line L517 (18.677953, -6.062663) -> (19.03857, -6.031611)
  line L518 (19.03857, -6.031611) -> (19.082004, -6.025325)
  line L519 (19.082004, -6.025325) -> (19.124295, -6.019229)
  line L520 (19.124295, -6.019229) -> (19.536918, -5.927217)
  line L521 (19.536918, -5.927217) -> (19.575971, -5.914835)
  line L522 (19.575971, -5.914835) -> (19.559588, -5.972747)
  line L523 (19.559588, -5.972747) -> (19.23288, -6.401562)
  line L524 (19.23288, -6.401562) -> (19.18335, -6.429566)
  line L525 (19.18335, -6.429566) -> (19.13363, -6.457378)
  line L526 (19.13363, -6.457378) -> (18.564225, -6.597968)
  line L527 (18.564225, -6.597968) -> (18.375059, -6.597968)
  line L528 (18.375059, -6.597968) -> (18.320195, -6.597968)
  line L529 (18.320195, -6.597968) -> (18.178653, -6.588633)
  line L530 (18.178653, -6.588633) -> (18.159222, -6.587681)
  line L531 (18.159222, -6.587681) -> (18.138458, -6.585776)
  line L532 (18.138458, -6.585776) -> (17.879949, -6.555486)
  line L533 (17.879949, -6.555486) -> (17.849088, -6.551676)
  line L534 (17.849088, -6.551676) -> (17.81175, -6.989826)
  line L535 (17.81175, -6.989826) -> (17.842992, -6.975158)
  line L536 (17.842992, -6.975158) -> (18.15103, -6.867716)
  line L537 (18.15103, -6.867716) -> (18.181892, -6.860667)
  line L538 (18.181892, -6.860667) -> (18.2118, -6.853238)
  line L539 (18.2118, -6.853238) -> (18.462879, -6.818376)
  line L540 (18.462879, -6.818376) -> (18.547842, -6.818376)
  line L541 (18.547842, -6.818376) -> (18.758345, -6.818376)
  line L542 (18.758345, -6.818376) -> (19.337274, -7.062026)
  line L543 (19.337274, -7.062026) -> (19.393091, -7.111746)
  line L544 (19.393091, -7.111746) -> (19.447955, -7.160133)
  line L545 (19.447955, -7.160133) -> (19.723799, -7.678293)
  line L546 (19.723799, -7.678293) -> (19.723799, -7.851839)
  line L547 (19.723799, -7.851839) -> (19.723799, -7.967472)
  line L548 (19.723799, -7.967472) -> (19.639979, -8.315896)
  line L549 (19.639979, -8.315896) -> (19.444716, -8.621649)
  line L550 (19.444716, -8.621649) -> (19.3889, -8.672322)
  line L551 (19.3889, -8.672322) -> (19.333083, -8.722042)
  line L552 (19.333083, -8.722042) -> (18.992088, -8.897684)
  line L553 (18.992088, -8.897684) -> (18.601563, -8.974074)
  line L554 (18.601563, -8.974074) -> (18.471452, -8.974074)
  line L555 (18.471452, -8.974074) -> (18.253139, -8.974074)
  line L556 (18.253139, -8.974074) -> (17.655731, -8.786051)
  line L557 (17.655731, -8.786051) -> (17.600866, -8.748712)
  line L558 (17.600866, -8.748712) -> (17.545241, -8.710613)
  line L559 (17.545241, -8.710613) -> (17.267301, -8.30561)
  line L560 (17.267301, -8.30561) -> (17.267301, -8.171116)
  line L561 (17.267301, -8.171116) -> (17.267301, -8.093583)
  line L562 (17.267301, -8.093583) -> (17.370361, -7.884795)
  line L563 (17.370361, -7.884795) -> (17.391126, -7.864221)
  line L564 (17.391126, -7.864221) -> (17.410938, -7.843647)
  line L565 (17.410938, -7.843647) -> (17.625822, -7.740205)
  line L566 (17.625822, -7.740205) -> (17.698212, -7.740205)
  line L567 (17.698212, -7.740205) -> (17.769459, -7.740205)
  line L568 (17.769459, -7.740205) -> (17.964722, -7.819835)
  line L569 (17.964722, -7.819835) -> (17.983391, -7.836217)
  line L570 (17.983391, -7.836217) -> (18.00206, -7.851839)
  line L571 (18.00206, -7.851839) -> (18.094071, -8.026337)
  line L572 (18.094071, -8.026337) -> (18.094071, -8.085391)
  line L573 (18.094071, -8.085391) -> (18.094071, -8.150542)
  line L574 (18.094071, -8.150542) -> (18.003012, -8.329041)
  line L575 (18.003012, -8.329041) -> (17.985677, -8.345805)
  line L576 (17.985677, -8.345805) -> (17.966817, -8.361426)
  line L577 (17.966817, -8.361426) -> (17.761268, -8.441817)
  line L578 (17.761268, -8.441817) -> (17.692878, -8.441817)
  line L579 (-20.470063, -8.89235) -> (-20.470063, -8.548497)
  line L580 (-20.470063, -8.548497) -> (-20.256132, -8.548497)
  line L581 (-20.256132, -8.548497) -> (-20.179646, -8.548497)
  line L582 (-20.179646, -8.548497) -> (-19.958475, -8.50392)
  line L583 (-19.958475, -8.50392) -> (-19.947103, -8.495538)
  line L584 (-19.947103, -8.495538) -> (-19.936777, -8.486203)
  line L585 (-19.936777, -8.486203) -> (-19.88199, -8.32085)
  line L586 (-19.88199, -8.32085) -> (-19.88199, -8.266176)
  line L587 (-19.88199, -8.266176) -> (-19.88199, -6.736461)
  line L588 (-19.88199, -6.736461) -> (-20.470063, -6.736461)
  line L589 (-20.470063, -6.736461) -> (-20.470063, -6.397562)
  line L590 (-20.470063, -6.397562) -> (-20.413218, -6.394514)
  line L591 (-20.413218, -6.394514) -> (-19.965695, -6.296216)
  line L592 (-19.965695, -6.296216) -> (-19.933653, -6.279642)
  line L593 (-19.933653, -6.279642) -> (-19.901611, -6.262116)
  line L594 (-19.901611, -6.262116) -> (-19.656685, -5.990463)
  line L595 (-19.656685, -5.990463) -> (-19.639121, -5.953125)
  line L596 (-19.639121, -5.953125) -> (-19.25153, -5.953125)
  line L597 (-19.25153, -5.953125) -> (-19.25153, -8.27532)
  line L598 (-19.25153, -8.27532) -> (-19.25153, -8.331136)
  line L599 (-19.25153, -8.331136) -> (-19.207086, -8.492681)
  line L600 (-19.207086, -8.492681) -> (-19.19779, -8.500872)
  line L601 (-19.19779, -8.500872) -> (-19.189522, -8.507921)
  line L602 (-19.189522, -8.507921) -> (-18.985992, -8.548497)
  line L603 (-18.985992, -8.548497) -> (-18.917793, -8.548497)
  line L604 (-18.917793, -8.548497) -> (-18.67281, -8.548497)
  line L605 (-18.67281, -8.548497) -> (-18.67281, -8.89235)
  line L606 (-18.67281, -8.89235) -> (-20.470063, -8.89235)
  line L607 (-16.940593, -8.581454) -> (-16.926115, -8.590788)
  line L608 (-16.926115, -8.590788) -> (-16.77943, -8.658987)
  line L609 (-16.77943, -8.658987) -> (-16.763809, -8.664131)
  line L610 (-16.763809, -8.664131) -> (-16.749331, -8.668322)
  line L611 (-16.749331, -8.668322) -> (-16.617124, -8.692134)
  line L612 (-16.617124, -8.692134) -> (-16.572547, -8.692134)
  line L613 (-16.572547, -8.692134) -> (-16.441293, -8.692134)
  line L614 (-16.441293, -8.692134) -> (-16.076485, -8.464486)
  line L615 (-16.076485, -8.464486) -> (-16.047529, -8.4201)
  line L616 (-16.047529, -8.4201) -> (-16.019716, -8.37457)
  line L617 (-16.019716, -8.37457) -> (-15.871888, -7.672959)
  line L618 (-15.871888, -7.672959) -> (-15.870936, -7.579043)
  line L619 (-15.870936, -7.579043) -> (-15.900844, -7.601521)
  line L620 (-15.900844, -7.601521) -> (-16.206787, -7.771067)
  line L621 (-16.206787, -7.771067) -> (-16.237839, -7.782496)
  line L622 (-16.237839, -7.782496) -> (-16.2687, -7.793736)
  line L623 (-16.2687, -7.793736) -> (-16.544734, -7.850695)
  line L624 (-16.544734, -7.850695) -> (-16.635603, -7.850695)
  line L625 (-16.635603, -7.850695) -> (-16.81753, -7.850695)
  line L626 (-16.81753, -7.850695) -> (-17.314735, -7.627429)
  line L627 (-17.314735, -7.627429) -> (-17.36217, -7.583043)
  line L628 (-17.36217, -7.583043) -> (-17.410747, -7.538466)
  line L629 (-17.410747, -7.538466) -> (-17.653635, -7.076504)
  line L630 (-17.653635, -7.076504) -> (-17.653635, -6.92258)
  line L631 (-17.653635, -6.92258) -> (-17.653635, -6.736461)
  line L632 (-17.653635, -6.736461) -> (-17.375695, -6.225921)
  line L633 (-17.375695, -6.225921) -> (-17.319879, -6.179439)
  line L634 (-17.319879, -6.179439) -> (-17.265015, -6.132957)
  line L635 (-17.265015, -6.132957) -> (-16.638841, -5.900547)
  line L636 (-16.638841, -5.900547) -> (-16.430053, -5.900547)
  line L637 (-16.430053, -5.900547) -> (-16.294608, -5.900547)
  line L638 (-16.294608, -5.900547) -> (-15.886366, -5.997512)
  line L639 (-15.886366, -5.997512) -> (-15.536989, -6.225921)
  line L640 (-15.536989, -6.225921) -> (-15.480221, -6.291072)
  line L641 (-15.480221, -6.291072) -> (-15.424404, -6.356033)
  line L642 (-15.424404, -6.356033) -> (-15.229141, -6.761416)
  line L643 (-15.229141, -6.761416) -> (-15.144369, -7.233666)
  line L644 (-15.144369, -7.233666) -> (-15.144369, -7.39159)
  line L645 (-15.144369, -7.39159) -> (-15.144369, -7.556945)
  line L646 (-15.144369, -7.556945) -> (-15.238285, -8.053197)
  line L647 (-15.238285, -8.053197) -> (-15.455455, -8.487347)
  line L648 (-15.455455, -8.487347) -> (-15.517368, -8.558784)
  line L649 (-15.517368, -8.558784) -> (-15.580423, -8.628888)
  line L650 (-15.580423, -8.628888) -> (-15.961805, -8.87711)
  line L651 (-15.961805, -8.87711) -> (-16.399954, -8.983409)
  line L652 (-16.399954, -8.983409) -> (-16.545687, -8.983409)
  line L653 (-16.545687, -8.983409) -> (-16.713136, -8.983409)
  line L654 (-16.713136, -8.983409) -> (-17.169956, -8.834628)
  line L655 (-17.169956, -8.834628) -> (-17.213389, -8.805672)
  line L656 (-17.213389, -8.805672) -> (-17.257966, -8.775764)
  line L657 (-17.257966, -8.775764) -> (-17.477041, -8.468868)
  line L658 (-17.477041, -8.468868) -> (-17.477041, -8.367522)
  line L659 (-17.477041, -8.367522) -> (-17.477041, -8.300276)
  line L660 (-17.477041, -8.300276) -> (-17.382934, -8.117396)
  line L661 (-17.382934, -8.117396) -> (-17.364265, -8.100822)
  line L662 (-17.364265, -8.100822) -> (-17.345787, -8.083296)
  line L663 (-17.345787, -8.083296) -> (-17.142142, -7.998333)
  line L664 (-17.142142, -7.998333) -> (-17.073943, -7.998333)
  line L665 (-17.073943, -7.998333) -> (-17.011841, -7.998333)
  line L666 (-17.011841, -7.998333) -> (-16.839247, -8.071866)
  line L667 (-16.839247, -8.071866) -> (-16.822674, -8.086154)
  line L668 (-16.822674, -8.086154) -> (-16.807244, -8.100822)
  line L669 (-16.807244, -8.100822) -> (-16.725519, -8.255889)
  line L670 (-16.725519, -8.255889) -> (-16.725519, -8.308467)
  line L671 (-16.725519, -8.308467) -> (-16.725519, -8.349996)
  line L672 (-16.725519, -8.349996) -> (-16.770096, -8.463534)
  line L673 (-16.770096, -8.463534) -> (-16.778287, -8.474774)
  line L674 (-16.778287, -8.474774) -> (-16.787622, -8.485251)
  line L675 (-16.787622, -8.485251) -> (-16.923068, -8.574024)
  line L676 (-16.923068, -8.574024) -> (-16.940593, -8.581454)
  line L677 (-15.909036, -6.866763) -> (-15.909036, -6.753035)
  line L678 (-15.909036, -6.753035) -> (-16.020669, -6.437757)
  line L679 (-16.020669, -6.437757) -> (-16.042386, -6.411849)
  line L680 (-16.042386, -6.411849) -> (-16.065246, -6.385179)
  line L681 (-16.065246, -6.385179) -> (-16.335946, -6.253925)
  line L682 (-16.335946, -6.253925) -> (-16.425862, -6.253925)
  line L683 (-16.425862, -6.253925) -> (-16.520922, -6.253925)
  line L684 (-16.520922, -6.253925) -> (-16.783431, -6.378893)
  line L685 (-16.783431, -6.378893) -> (-16.805148, -6.404801)
  line L686 (-16.805148, -6.404801) -> (-16.828008, -6.429566)
  line L687 (-16.828008, -6.429566) -> (-16.936402, -6.737604)
  line L688 (-16.936402, -6.737604) -> (-16.936402, -6.840855)
  line L689 (-16.936402, -6.840855) -> (-16.936402, -6.951345)
  line L690 (-16.936402, -6.951345) -> (-16.819626, -7.260526)
  line L691 (-16.819626, -7.260526) -> (-16.795813, -7.286434)
  line L692 (-16.795813, -7.286434) -> (-16.773144, -7.3112)
  line L693 (-16.773144, -7.3112) -> (-16.487965, -7.439216)
  line L694 (-16.487965, -7.439216) -> (-16.391763, -7.439216)
  line L695 (-16.391763, -7.439216) -> (-16.303943, -7.439216)
  line L696 (-16.303943, -7.439216) -> (-16.061055, -7.310247)
  line L697 (-16.061055, -7.310247) -> (-16.039338, -7.284149)
  line L698 (-16.039338, -7.284149) -> (-16.017621, -7.258621)
  line L699 (-16.017621, -7.258621) -> (-15.909036, -6.963918)
  line L700 (-15.909036, -6.963918) -> (-15.909036, -6.866763)
  line L701 (-29.911357, 16.940403) -> (-28.194667, 16.119919)
  line L702 (-28.194667, 16.119919) -> (-28.483008, 15.517368)
  line L703 (-28.483008, 15.517368) -> (-28.579134, 15.56385)
  line L704 (-28.579134, 15.56385) -> (-29.008045, 15.702534)
  line L705 (-29.008045, 15.702534) -> (-29.370814, 15.721012)
  line L706 (-29.370814, 15.721012) -> (-29.433869, 15.706534)
  line L707 (-29.433869, 15.706534) -> (-29.496906, 15.693199)
  line L708 (-29.496906, 15.693199) -> (-29.769759, 15.530703)
  line L709 (-29.769759, 15.530703) -> (-29.98992, 15.24762)
  line L710 (-29.98992, 15.24762) -> (-30.025048, 15.172182)
  line L711 (-30.025048, 15.172182) -> (-30.05709, 15.103983)
  line L712 (-30.05709, 15.103983) -> (-27.229365, 13.752195)
  line L713 (-27.229365, 13.752195) -> (-27.191094, 13.734478)
  line L714 (-27.191094, 13.734478) -> (-26.930661, 13.63218)
  line L715 (-26.930661, 13.63218) -> (-26.916202, 13.629132)
  line L716 (-26.916202, 13.629132) -> (-26.902753, 13.628179)
  line L717 (-26.902753, 13.628179) -> (-26.792149, 13.661136)
  line L718 (-26.792149, 13.661136) -> (-26.7839, 13.669518)
  line L719 (-26.7839, 13.669518) -> (-26.773556, 13.678662)
  line L720 (-26.773556, 13.678662) -> (-26.665028, 13.817346)
  line L721 (-26.665028, 13.817346) -> (-26.653674, 13.834872)
  line L722 (-26.653674, 13.834872) -> (-26.642301, 13.85335)
  line L723 (-26.642301, 13.85335) -> (-26.462469, 14.188249)
  line L724 (-26.462469, 14.188249) -> (-26.437666, 14.237017)
  line L725 (-26.437666, 14.237017) -> (-25.867157, 13.96384)
  line L726 (-25.867157, 13.96384) -> (-27.129105, 11.324463)
  line L727 (-27.129105, 11.324463) -> (-27.699595, 11.597259)
  line L728 (-27.699595, 11.597259) -> (-27.68306, 11.632311)
  line L729 (-27.68306, 11.632311) -> (-27.552834, 11.935015)
  line L730 (-27.552834, 11.935015) -> (-27.542509, 11.961114)
  line L731 (-27.542509, 11.961114) -> (-27.533194, 11.987974)
  line L732 (-27.533194, 11.987974) -> (-27.474272, 12.213145)
  line L733 (-27.474272, 12.213145) -> (-27.471186, 12.231624)
  line L734 (-27.471186, 12.231624) -> (-27.470157, 12.243054)
  line L735 (-27.470157, 12.243054) -> (-27.514601, 12.347638)
  line L736 (-27.514601, 12.347638) -> (-27.524926, 12.356782)
  line L737 (-27.524926, 12.356782) -> (-27.53527, 12.367069)
  line L738 (-27.53527, 12.367069) -> (-27.772976, 12.503658)
  line L739 (-27.772976, 12.503658) -> (-27.8102, 12.521184)
  line L740 (-27.8102, 12.521184) -> (-27.898039, 12.563475)
  line L741 (-27.898039, 12.563475) -> (-30.645144, 13.877163)
  line L742 (-30.645144, 13.877163) -> (-30.676158, 13.812012)
  line L743 (-30.676158, 13.812012) -> (-30.712334, 13.736574)
  line L744 (-30.712334, 13.736574) -> (-30.750586, 13.066966)
  line L745 (-30.750586, 13.066966) -> (-30.721649, 13.007911)
  line L746 (-30.721649, 13.007911) -> (-30.693722, 12.949999)
  line L747 (-30.693722, 12.949999) -> (-30.075683, 12.431268)
  line L748 (-30.075683, 12.431268) -> (-29.980604, 12.385929)
  line L749 (-29.980604, 12.385929) -> (-30.26584, 11.788521)
  line L750 (-30.26584, 11.788521) -> (-31.98255, 12.609957)
  line L751 (-31.98255, 12.609957) -> (-29.911357, 16.940403)
  line L752 (-23.801127, 17.377791) -> (-24.286902, 17.804701)
  line L753 (-24.286902, 17.804701) -> (-24.107051, 18.009108)
  line L754 (-24.107051, 18.009108) -> (-24.076057, 18.045303)
  line L755 (-24.076057, 18.045303) -> (-23.917904, 18.332767)
  line L756 (-23.917904, 18.332767) -> (-23.918951, 18.351246)
  line L757 (-23.918951, 18.351246) -> (-24.097755, 18.597372)
  line L758 (-24.097755, 18.597372) -> (-24.132883, 18.628233)
  line L759 (-24.132883, 18.628233) -> (-26.226821, 20.465034)
  line L760 (-26.226821, 20.465034) -> (-26.262997, 20.497038)
  line L761 (-26.262997, 20.497038) -> (-26.531697, 20.64277)
  line L762 (-26.531697, 20.64277) -> (-26.54928, 20.639532)
  line L763 (-26.54928, 20.639532) -> (-26.566863, 20.637436)
  line L764 (-26.566863, 20.637436) -> (-26.813847, 20.445222)
  line L765 (-26.813847, 20.445222) -> (-26.84486, 20.409217)
  line L766 (-26.84486, 20.409217) -> (-27.023663, 20.20443)
  line L767 (-27.023663, 20.20443) -> (-27.510467, 20.630388)
  line L768 (-27.510467, 20.630388) -> (-24.29618, 24.296179)
  line L769 (-24.29618, 24.296179) -> (-22.881298, 23.056024)
  line L770 (-22.881298, 23.056024) -> (-23.307084, 22.570249)
  line L771 (-23.307084, 22.570249) -> (-23.368083, 22.610445)
  line L772 (-23.368083, 22.610445) -> (-23.855915, 22.878288)
  line L773 (-23.855915, 22.878288) -> (-23.892091, 22.891814)
  line L774 (-23.892091, 22.891814) -> (-23.929296, 22.906101)
  line L775 (-23.929296, 22.906101) -> (-24.267243, 22.958679)
  line L776 (-24.267243, 22.958679) -> (-24.297208, 22.955821)
  line L777 (-24.297208, 22.955821) -> (-24.328222, 22.953726)
  line L778 (-24.328222, 22.953726) -> (-24.636222, 22.832758)
  line L779 (-24.636222, 22.832758) -> (-24.666207, 22.811041)
  line L780 (-24.666207, 22.811041) -> (-24.697182, 22.790467)
  line L781 (-24.697182, 22.790467) -> (-25.155049, 22.336696)
  line L782 (-25.155049, 22.336696) -> (-25.216028, 22.266211)
  line L783 (-25.216028, 22.266211) -> (-25.636671, 21.786913)
  line L784 (-25.636671, 21.786913) -> (-24.581434, 20.860893)
  line L785 (-24.581434, 20.860893) -> (-24.500834, 20.952523)
  line L786 (-24.500834, 20.952523) -> (-24.45639, 21.00453)
  line L787 (-24.45639, 21.00453) -> (-24.251755, 21.43125)
  line L788 (-24.251755, 21.43125) -> (-24.255889, 21.465349)
  line L789 (-24.255889, 21.465349) -> (-24.261051, 21.500592)